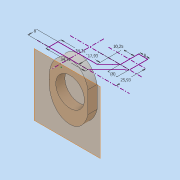
# Autodesk Inventor part: lw_4_2_крепление_yjdjt
Saved by Autodesk Inventor 2019 (Build 230136000, 136)
## iProperties
Created: 2021-03-07
Part Number: lw_4_2_крепление_yjdjt
Material: Типовые
Document SubType Name: Modeling
Designer: Kurbatova
Density: 1 g/cm^3
Appearance: По умолчанию
Author: Kurbatova
Autodesk Inventor part; units mm, degrees
ref_plane "YZ Plane" through (0, 0, 0) normal (1, 0, 0) x (0, 1, 0)
sketch "Основной эскиз" plane through (0, 0, 0) normal (0, 1, 0) x (-1, 0, 0)
  line L0 (21.0127, -18.1102) -> (-13.2973, -18.1102)
  line L1 (21.0127, -18.1102) -> (21.0127, -10.1102)
  line L2 (21.0127, -10.1102) -> (-13.2973, -10.1102)
  line L3 (20.451, -28.0402) -> (-43.6243, -28.0402)
  line L4 (-23.5473, -28.0402) -> (-23.5473, -44.0402)
  line L5 (-23.5473, -44.0402) -> (-31.5473, -44.0402)
  line L6 (-31.5473, -44.0402) -> (-31.5473, -28.0402)
  line L7 (-31.5473, -28.0402) -> (-13.2973, -10.1102)
  line L8 (-23.5473, -28.0402) -> (-13.2973, -18.1102)
  line L9 (-5.2293, -36.0402) -> (-38.0765, -36.0402)
  line L10 (31.3847, -10.1102) -> (-49.5844, -10.1102)
  line L11 (3.1555, -40.2525) -> (3.1555, 5.5167)
  point P0 (0, 0)
  point P1 (-23.5473, -36.0402)
  dimension "d0" = 34.31
  dimension "d2" = 8
  dimension "d3" = 34.31
  dimension "d5" = 8
  dimension "d7" = 17.93
  dimension "d8" = 25.93
  dimension "d9" = 10.25
  dimension "d10" = 8
  constraints: 24 end point, 4 perpendicular, 4 point on line, 3 horizontal, 3 vertical, 1 midpoint
  measures "d0" distance of L0.start L0.end
  measures "d2" distance of L0.start L1.end
  measures "d3" distance of L1.end L2.end
  measures "d5" distance of L4.end L5.end
  measures "d7" vertical distance of L6.end L2.end
  measures "d8" distance between parallel lines of L10 L9
  measures "d9" distance from line of L0.end L4
  measures "d10" distance of L6.end L4.start
extrude "ВыдавливаниеОсновной" add sketch "Основной эскиз" against normal blind 49.49 contours L0 L11 L2 L1 | L0 L8 L3 L7 L2 L11 | L4 L9 L6 L3 | L4 L5 L6 L9
ref_plane "РабПлоскость18" through (13.2973, 0, -18.1102) normal (0, 0, -1) x (-1, 0, 0)
ref_plane "РабПлоскость41" through (13.0446, -16.4427, -18.1102) normal (0.6958, 0.0022, 0.7182) x (0.0031, -1, 0)
sketch "Ручка" plane through (13.0446, -16.4427, -18.1102) normal (0.6958, 0.0022, 0.7182) x (0.0031, -1, 0)
  arc A0 (13.7315, 14.434) -> (17.6656, 0.1628) centre (18.6248, 8.105) ccw
  arc A1 (14.1675, 14.7411) -> (13.7315, 14.434) centre (17.4015, 9.6873) ccw
  arc A2 (-1.0594, 0.1628) -> (2.3115, 14.434) centre (-2.4886, 8.0341) ccw
  line L0 (2.3115, 14.434) -> (13.7315, 14.434)
  line L1 (-1.0594, 0.1628) -> (17.6656, 0.1628)
  line L2 (17.728, 0.1415) -> (-1.1219, 0.184) projected
  point P0 (-16.4836, -21.933)
  point P1 (-16.4096, 14.4897)
  point P2 (12.9792, 13.7423)
  point P3 (8.3031, 0.1628)
  dimension "d341" = 16
  dimension "d345" = 12
  dimension "d352" = 11.42
  dimension "d353" = 14.2712
  constraints: 7 point on circle, 4 end point, 3 centre point, 2 horizontal, 2 midpoint, 1 tangent
  measures "d341" diameter of A0
  measures "d345" diameter of A1
  measures "d352" distance of L0.start L0.end
  measures "d353" distance between parallel lines of L1 L0
extrude "Выдавливание32" [suppressed]
sketch "Отвертстия" plane through (13.2973, 0, -18.1102) normal (0, 0, -1) x (-1, 0, 0)
  line L0 (48.4897, -24.745) -> (-16.3078, -24.745)
  line L1 (0, 0) -> (34.31, 0) projected
  line L2 (34.31, -49.49) -> (0, -49.49) projected
  line L3 (34.31, 0) -> (34.31, -49.49) projected
  circle A0 centre (15.6477, -24.745) radius 12.5
  ellipse E0 centre (15.7193, -26.6222) end of major axis (16.7788, -49.3596) minor radius 18.1572 (16.4021, -49.3722) -> (33.79, -24.745) ccw
  ellipse E1 centre (15.7193, -22.8678) end of major axis (16.7788, -0.1304) minor radius 18.1572 (33.79, -24.745) -> (16.4021, -0.1178) ccw
  ellipse E2 centre (15.7193, -26.6222) end of major axis (14.6417, -49.4193) minor radius 16.4679 (0, -34.17) -> (16.4021, -49.3722) ccw
  ellipse E3 centre (15.7193, -22.8678) end of major axis (14.6417, -0.0707) minor radius 16.4679 (16.4021, -0.1178) -> (0, -15.32) ccw
  line L4 (0, -34.17) -> (0, -15.32)
  line L5 (0, 0) -> (0, -49.49) projected
  line L6 (16.4339, -64.2485) -> (15.7511, 14.4026)
  point P0 (17.155, 0)
  point P1 (0, -24.745)
  point P2 (16.091, -24.745)
  dimension "d31" = 25
  dimension "d329" = 18.85
  constraints: 6 end point, 4 midpoint, 4 symmetric about line, 3 horizontal, 3 point on line, 1 centre point, 1 collinear, 16 other
  measures "d31" diameter of A0
  measures "d329" distance of L4.start L4.end
extrude "Корпус элипса" add sketch "Отвертстия" against normal blind 8 separate body contours E0 E2 L6 A0 L0 | L0 A0 L6 E3 E1 | A0 L0 L4 E3 L6 | L6 E2 L4 L0 A0
sketch "Эскиз42" plane through (13.2973, 0, -18.1102) normal (0, 0, -1) x (-1, 0, 0)
  ellipse E0 centre (9.8832, -41.1273) end of major axis (6.418, -38.906) minor radius 3.115
  line L0 (48.3173, -24.7445) -> (-16.4639, -24.7445) projected
  ellipse E1 centre (9.8832, -8.3617) end of major axis (6.418, -10.5829) minor radius 3.115
  line L1 (15.9267, -61.1755) -> (15.9267, 11.6866)
  ellipse E2 centre (21.9702, -41.1273) end of major axis (25.4354, -38.906) minor radius 3.115
  ellipse E3 centre (21.9702, -8.3617) end of major axis (25.4354, -10.5829) minor radius 3.115
  point P0 (13.2973, 0)
  point P1 (15.9267, -24.7445)
  dimension "d401" = 4.116
  dimension "d402" = 3.115
  constraints: 3 symmetric about line, 3 vertical, 2 end point, 2 midpoint, 9 other
extrude "Дырки" cut sketch "Эскиз42" against normal blind 3
